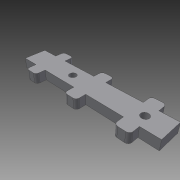
# Autodesk Inventor part: rope_mount_holder
Saved by Autodesk Inventor 2014 (Build 180170000, 170)
## iProperties
Created: 2013-12-17
Part Number: rope_mount_holder
Material: Generic
Document SubType Name: Modeling
Designer: buben
Density: 1 g/cm^3
Appearance: Anodized - Dark Gray
Author: buben
Autodesk Inventor part; units mm, degrees
ref_plane "YZ Plane" through (0, 0, 0) normal (1, 0, 0) x (0, 1, 0)
ref_plane "XZ Plane" through (0, 0, 0) normal (0, 1, 0) x (-1, 0, 0)
ref_plane "XY Plane" through (0, 0, 0) normal (0, 0, 1) x (1, 0, 0)
sketch "Sketch1" plane through (0, 0, 0) normal (0, 0, 1) x (1, 0, 0)
  line L0 (0, 0) -> (88.1, 0)
  line L1 (88.1, 0) -> (88.1, 13.5)
  line L2 (88.1, 13.5) -> (0, 13.5)
  line L3 (0, 13.5) -> (0, 0)
  dimension "d0" = 88.1
  dimension "d1" = 13.5
  constraints: 8 end point, 2 parallel, 1 horizontal, 1 perpendicular
  measures "d0" distance of L0.start L0.end
  measures "d1" distance of L2.end L0.start
extrude "Extrusion1" add sketch "Sketch1" along normal blind 6
sketch "Sketch2" plane through (0, 0, 6) normal (0, 0, 1) x (1, 0, 0)
  line L0 (0, 0) -> (88.1, 0) projected
  line L1 (88.1, 13.5) -> (0, 13.5) projected
  line L2 (40.05, 13.5) -> (48.05, 13.5)
  line L3 (48.05, 13.5) -> (48.05, 17.5)
  line L4 (46.05, 19.5) -> (42.05, 19.5)
  line L5 (40.05, 17.5) -> (40.05, 13.5)
  line L6 (70.05, 13.5) -> (78.05, 13.5)
  line L7 (78.05, 13.5) -> (78.05, 17.5)
  line L8 (76.05, 19.5) -> (72.05, 19.5)
  line L9 (70.05, 17.5) -> (70.05, 13.5)
  line L10 (10.05, 13.5) -> (18.05, 13.5)
  line L11 (18.05, 13.5) -> (18.05, 17.5)
  line L12 (16.05, 19.5) -> (12.05, 19.5)
  line L13 (10.05, 17.5) -> (10.05, 13.5)
  line L14 (10.05, 0) -> (18.05, 0)
  line L15 (18.05, 0) -> (18.05, -4)
  line L16 (16.05, -6) -> (12.05, -6)
  line L17 (10.05, -4) -> (10.05, 0)
  line L18 (40.05, 0) -> (48.05, 0)
  line L19 (48.05, 0) -> (48.05, -4)
  line L20 (46.05, -6) -> (42.05, -6)
  line L21 (40.05, -4) -> (40.05, 0)
  line L22 (70.05, 0) -> (78.05, 0)
  line L23 (78.05, 0) -> (78.05, -4)
  line L24 (76.05, -6) -> (72.05, -6)
  line L25 (70.05, -4) -> (70.05, 0)
  arc A0 (12.05, 19.5) -> (10.05, 17.5) centre (12.05, 17.5) ccw
  arc A1 (18.05, 17.5) -> (16.05, 19.5) centre (16.05, 17.5) ccw
  arc A2 (42.05, 19.5) -> (40.05, 17.5) centre (42.05, 17.5) ccw
  arc A3 (48.05, 17.5) -> (46.05, 19.5) centre (46.05, 17.5) ccw
  arc A4 (72.05, 19.5) -> (70.05, 17.5) centre (72.05, 17.5) ccw
  arc A5 (78.05, 17.5) -> (76.05, 19.5) centre (76.05, 17.5) ccw
  arc A6 (70.05, -4) -> (72.05, -6) centre (72.05, -4) ccw
  arc A7 (76.05, -6) -> (78.05, -4) centre (76.05, -4) ccw
  arc A8 (40.05, -4) -> (42.05, -6) centre (42.05, -4) ccw
  arc A9 (46.05, -6) -> (48.05, -4) centre (46.05, -4) ccw
  arc A10 (16.05, -6) -> (18.05, -4) centre (16.05, -4) ccw
  arc A11 (10.05, -4) -> (12.05, -6) centre (12.05, -4) ccw
  line L26 (88.1, 13.5) -> (0, 13.5) projected
  line L27 (18.05, 15.5) -> (40.05, 15.5) construction
  line L28 (48.05, 15.5) -> (70.05, 15.5) construction
  point P0 (44.05, 19.5)
  point P1 (44.05, 13.5)
  dimension "d4" = 2
  dimension "d5" = 8
  dimension "d6" = 8
  dimension "d7" = 8
  dimension "d8" = 6
  dimension "d9" = 6
  dimension "d10" = 22
  constraints: 52 end point, 24 point on circle, 24 tangent, 12 centre point, 12 parallel, 11 collinear, 11 equal radius, 6 horizontal, 6 midpoint, 6 perpendicular, 6 point on line, 1 vertical alignment
  measures "d4" radius of A0
  measures "d5" distance between parallel lines of L11 L13
  measures "d6" distance between parallel lines of L3 L5
  measures "d7" distance between parallel lines of L7 L9
  measures "d8" distance between parallel lines of L1 L12
  measures "d9" distance between parallel lines of L0 L16
  measures "d10" distance of L27.start L27.end
extrude "Extrusion2" add sketch "Sketch2" against normal blind 6
sketch "Sketch3" plane through (0, 0, 6) normal (0, 0, 1) x (1, 0, 0)
  line L0 (0, 13.5) -> (0, 0) projected
  circle A0 centre (31.889, 6.75) radius 2.25
  circle A1 centre (75.859, 6.75) radius 2.25
  point P0 (0, 6.75)
  dimension "d13" = 31.889
  dimension "d14" = 75.859
  dimension "d15" = 4.5
  constraints: 2 centre point, 2 horizontal alignment, 1 equal radius, 1 midpoint
  measures "d13" horizontal distance of L0.start A0.centre
  measures "d14" distance from line of L0 A1.centre
  measures "d15" diameter of A0
extrude "Extrusion3" cut sketch "Sketch3" against normal through all
body "Solid1"
